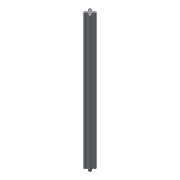
# Autodesk Inventor part: 20x20extrusion
Saved by Autodesk Inventor 2015 (Build 190159000, 159)
## iProperties
Created: 2015-01-22
Part Number: 20x20extrusion
Material: Generic
Document SubType Name: Modeling
Designer: rihoobler
Density: 1 g/cm^3
Appearance: Default
Author: rihoobler
Autodesk Inventor part; units mm, degrees
ref_plane "YZ Plane" through (0, 0, 0) normal (1, 0, 0) x (0, 1, 0)
ref_plane "XZ Plane" through (0, 0, 0) normal (0, 1, 0) x (-1, 0, 0)
ref_plane "XY Plane" through (0, 0, 0) normal (0, 0, 1) x (1, 0, 0)
sketch "Sketch1" plane through (0, 0, 0) normal (0, 1, 0) x (-1, 0, 0)
  line L0 (0, 0) -> (20, 0)
  line L1 (20, 0) -> (20, 20)
  line L2 (20, 20) -> (0, 20)
  line L3 (0, 20) -> (0, 0)
  line L4 (6, 0) -> (14, 0)
  line L5 (14, 0) -> (14, 4)
  line L6 (14, 4) -> (6, 4)
  line L7 (6, 4) -> (6, 0)
  line L8 (0, 6) -> (4, 6)
  line L9 (4, 6) -> (4, 14)
  line L10 (4, 14) -> (0, 14)
  line L11 (0, 14) -> (0, 6)
  line L12 (6, 20) -> (14, 20)
  line L13 (14, 20) -> (14, 16)
  line L14 (14, 16) -> (6, 16)
  line L15 (6, 16) -> (6, 20)
  line L16 (20, 14) -> (16, 14)
  line L17 (16, 14) -> (16, 6)
  line L18 (16, 6) -> (20, 6)
  line L19 (20, 6) -> (20, 14)
  dimension "d0" = 20
  dimension "d1" = 20
  dimension "d2" = 8
  dimension "d3" = 6
  dimension "d4" = 8
  dimension "d5" = 6
  dimension "d6" = 4
  dimension "d7" = 4
  dimension "d8" = 4
  dimension "d9" = 4
  constraints: 40 end point, 10 parallel, 8 point on line, 5 horizontal, 5 perpendicular
  measures "d0" distance of L2.end L1.end
  measures "d1" distance of L1.end L0.end
  measures "d2" distance between parallel lines of L5 L7
  measures "d3" distance between parallel lines of L1 L5
  measures "d4" distance between parallel lines of L8 L10
  measures "d5" distance between parallel lines of L0 L8
  measures "d6" distance between parallel lines of L11 L9
  measures "d7" distance between parallel lines of L12 L14
  measures "d8" distance between parallel lines of L1 L17
  measures "d9" distance between parallel lines of L0 L6
extrude "Extrusion1" add sketch "Sketch1" along normal blind 381 contours L3 L8 L9 L10 L2 L15 L14 L13 L1 L16 L17 L18 L0 L5 L6 L7
fillet "Fillet1" radius 1.27 12 edges at (0, 190.5, 20) (0, 190.5, 14) (-6, 190.5, 20) (-14, 190.5, 20) (-20, 190.5, 20) (-20, 190.5, 14) (0, 190.5, 6) (0, 190.5, 0) (-6, 190.5, 0) (-14, 190.5, 0) (-20, 190.5, 0) (-20, 190.5, 6)
body "Solid1"
